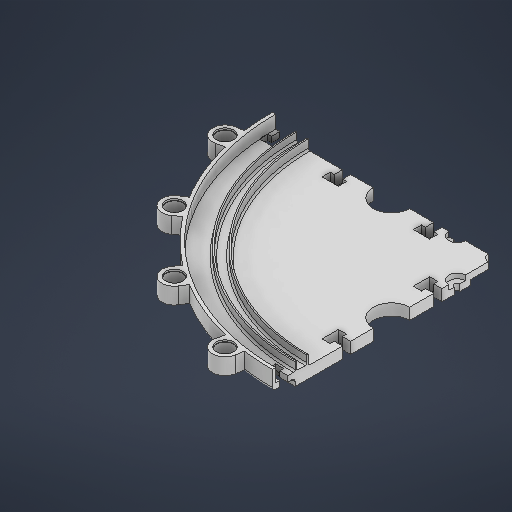
# Autodesk Inventor part: Base_frame_v2
Saved by Autodesk Inventor 2026 (Build 300175050, 175E)
## iProperties
Created: 2026-04-30
Part Number: Base_frame_v2
Material: Generic
Document SubType Name: Modeling
Designer: sniel
Density: 1 g/cm^3
Appearance: Default
Author: sniel
Autodesk Inventor part; units mm, degrees
ref_plane "YZ Plane" through (0, 0, 0) normal (1, 0, 0) x (0, 1, 0)
ref_plane "XZ Plane" through (0, 0, 0) normal (0, 1, 0) x (-1, 0, 0)
ref_plane "XY Plane" through (0, 0, 0) normal (0, 0, 1) x (1, 0, 0)
sketch "Sketch1" plane through (0, 0, 0) normal (1, 0, 0) x (0, 1, 0)
  line L0 (0, 122.235526) -> (11, 122.235526)
  line L1 (5, 0) -> (0, 0)
  line L2 (11, 122.235526) -> (11, 114.235526)
  line L3 (5, 0) -> (5, 114.235526)
  line L4 (11, 118.235526) -> (11, 115.085526)
  line L5 (11, 118.235526) -> (11, 121.385526)
  line L6 (11, 118.235526) -> (6, 118.235526)
  line L7 (6, 118.235526) -> (6, 115.085526)
  line L8 (6, 115.085526) -> (11, 115.085526)
  line L9 (6, 118.235526) -> (6, 121.385526)
  line L10 (6, 121.385526) -> (11, 121.385526)
  line L11 (5, 0) -> (-2, 0)
  line L12 (-2, 0) -> (-2, 122.235526)
  line L13 (-2, 122.235526) -> (0, 122.235526)
  line L14 (5, 114.235526) -> (11, 114.235526)
  line L15 (11, 118.235526) -> (12, 118.235526)
  line L16 (12, 118.235526) -> (12, 134.235526)
  line L17 (6, 118.235526) -> (6, 134.235526)
  line L18 (6, 134.235526) -> (12, 134.235526)
  line L19 (12, 134.235526) -> (14, 134.235526)
  line L20 (14, 134.235526) -> (14, 136.235526)
  line L21 (6, 118.235526) -> (2.5, 118.235526)
  line L22 (2.5, 118.235526) -> (2.5, 134.235526)
  line L23 (2.5, 134.235526) -> (2.5, 136.235526)
  line L24 (2.5, 136.235526) -> (14, 136.235526)
  point P0 (2.5, 122.235526)
  point P1 (6, 122.235526)
  dimension "d0" = 8
  dimension "d1" = 3.15
  dimension "d2" = 3.15
  dimension "d3" = 5
  dimension "d12" = 7
  dimension "d16" = 1
  dimension "d17" = 16
  dimension "d18" = 16
  dimension "d19" = 2
  dimension "d20" = 2
  dimension "d21" = 3.5
  dimension "d22" = 16
  dimension "d23" = 2
  constraints: 50 end point, 4 horizontal, 4 perpendicular, 4 point on line, 3 vertical, 1 midpoint
  measures "d0" distance of L0.end L2.end
  measures "d1" distance of L4.start L4.end
  measures "d2" distance of L4.start L5.end
  measures "d3" distance of L4.start L6.end
  measures "d12" distance of L1.start L11.end
  measures "d16" distance of L4.start L15.end
  measures "d17" distance of L15.end L16.end
  measures "d18" distance of L6.end L17.end
  measures "d19" distance of L16.end L19.end
  measures "d20" distance of L19.end L20.end
  measures "d21" distance of L6.end L21.end
  measures "d22" distance of L21.end L22.end
  measures "d23" distance of L22.end L23.end
revolve "Revolution1" add sketch "Sketch1" angle 360 about axis through (0, 5, 0) along (0, -1, 0) contours L0 L22 L21 L7 L8 L2 L14 L3 L1 L11 L12 L13 | L22 L23 L24 L20 L19 L18 L17 L0 | L0 L17 L9 L21 L22 | L0 L2 L10 L17
sketch "Sketch5" plane through (0, 5, 0) normal (0, 1, 0) x (1, 0, 0)
  circle A0 centre (0, 0) radius 4.1
  line L0 (0, 0) -> (0, -63.331)
  line L1 (0, 0) -> (-63.331, 0)
  circle A1 centre (0, -63.331) radius 11.1
  circle A2 centre (-63.331, 0) radius 11.1
  line L2 (0, 0) -> (0, 63.331)
  circle A3 centre (0, 63.331) radius 11.1
  line L3 (0, 0) -> (0, 35)
  line L4 (0, 35) -> (0, 37.5)
  line L5 (0, 35) -> (0, 32.5)
  line L6 (0, 32.5) -> (-5, 32.5)
  line L7 (-5, 32.5) -> (-5, 30)
  line L8 (-5, 30) -> (-10, 30)
  line L9 (-10, 30) -> (-10, 40)
  line L10 (-10, 40) -> (-5, 40)
  line L11 (-5, 40) -> (-5, 37.5)
  line L12 (-5, 37.5) -> (0, 37.5)
  line L13 (0, 0) -> (-132, 132)
  line L14 (0, 0) -> (186.67619, 0) construction
  line L15 (-32.5, 0) -> (-32.5, 5)
  line L16 (-32.5, 5) -> (-30, 5)
  line L17 (-30, 5) -> (-30, 10)
  line L18 (-30, 10) -> (-40, 10)
  line L19 (-40, 10) -> (-40, 5)
  line L20 (-40, 5) -> (-37.5, 5)
  line L21 (-37.5, 5) -> (-37.5, 0)
  line L22 (0, 0) -> (-178, 0)
  line L23 (0, -32.5) -> (-5, -32.5)
  line L24 (-5, -32.5) -> (-5, -30)
  line L25 (-5, -30) -> (-10, -30)
  line L26 (-10, -30) -> (-10, -40)
  line L27 (-10, -40) -> (-5, -40)
  line L28 (-5, -37.5) -> (0, -37.5)
  line L29 (-40, -10) -> (-40, -5)
  line L30 (-40, -5) -> (-37.5, -5)
  line L31 (-32.5, -5) -> (-30, -5)
  line L32 (-30, -5) -> (-30, -10)
  line L33 (-32.5, 0) -> (-32.5, -5)
  line L34 (-30, -10) -> (-40, -10)
  line L35 (-37.5, -5) -> (-37.5, 0)
  line L36 (-5, -37.5) -> (-5, -40)
  line L37 (0, -63.331) -> (0, -88.331)
  line L38 (-10, -85.831) -> (-10, -95.831)
  line L39 (-10, -95.831) -> (-5, -95.831)
  line L40 (0, -88.331) -> (-5, -88.331)
  line L41 (-5, -88.331) -> (-5, -85.831)
  line L42 (-5, -93.331) -> (0, -93.331)
  line L43 (-5, -85.831) -> (-10, -85.831)
  line L44 (-5, -93.331) -> (-5, -95.831)
  line L45 (-63.331, 0) -> (-88.331, 0)
  line L46 (-85.831, -5) -> (-85.831, -10)
  line L47 (-88.331, -5) -> (-85.831, -5)
  line L48 (-88.331, 0) -> (-88.331, -5)
  line L49 (-93.331, -5) -> (-93.331, 0)
  line L50 (-85.831, -10) -> (-95.831, -10)
  line L51 (-95.831, -10) -> (-95.831, -5)
  line L52 (-95.831, -5) -> (-93.331, -5)
  line L53 (0, -88.331) -> (0, -93.331)
  line L54 (-93.331, 0) -> (-88.331, 0)
  point P0 (-37.5, 0)
  point P1 (-37.5, 0)
  point P2 (0, -37.5)
  dimension "d13" = 8.2
  dimension "d32" = 63.331
  dimension "d33" = 63.331
  dimension "d34" = 22.2
  dimension "d35" = 22.2
  dimension "d36" = 63.331
  dimension "d37" = 22.2
  dimension "d44" = 35
  dimension "d45" = 2.5
  dimension "d46" = 2.5
  dimension "d47" = 5
  dimension "d48" = 2.5
  dimension "d49" = 10
  dimension "d50" = 5
  dimension "d51" = 135
  dimension "d52" = 25
  dimension "d53" = 25
  constraints: 110 end point, 22 symmetric about line, 16 point on line, 6 perpendicular, 6 vertical, 4 centre point, 4 coincident, 3 horizontal, 1 equal length
  measures "d13" diameter of A0
  measures "d32" distance of L0.start L0.end
  measures "d33" distance of L0.start L1.end
  measures "d34" diameter of A1
  measures "d35" diameter of A2
  measures "d36" distance of L0.start L2.end
  measures "d37" diameter of A3
  measures "d44" distance of L0.start L3.end
  measures "d45" distance of L3.end L4.end
  measures "d46" distance of L3.end L5.end
  measures "d47" distance of L5.end L6.end
  measures "d48" distance of L6.end L7.end
  measures "d49" distance of L8.end L9.end
  measures "d50" distance of L9.end L10.end
  measures "d51" angle of L14 L13
  measures "d52" distance of L37.start L37.end
  measures "d53" distance of L45.start L45.end
extrude "Extrusion4" cut sketch "Sketch5" against normal blind 10
sketch "Sketch2" plane through (0, 0, 0) normal (1, 0, 0) x (0, 1, 0)
  line L0 (88, 190) -> (-72, 190)
  line L1 (-72, 190) -> (-72, -189)
  line L2 (-72, -189) -> (88, -189)
  line L3 (88, -189) -> (88, 190)
  point P0 (0, 0)
  constraints: 8 end point, 2 parallel, 1 horizontal, 1 perpendicular
extrude "Extrusion1" cut sketch "Sketch2" along normal blind 183.5
sketch "Sketch3" plane through (0, 0, 0) normal (0, 0, 1) x (1, 0, 0)
  line L0 (129, 60) -> (-156, 60)
  line L1 (-156, 60) -> (-156, -67)
  line L2 (-156, -67) -> (129, -67)
  line L3 (129, -67) -> (129, 60)
  point P0 (0, 0)
  constraints: 8 end point, 2 parallel, 1 horizontal, 1 perpendicular
extrude "Extrusion2" cut sketch "Sketch3" against normal blind 183.5
fillet "Fillet1" radius 2 2 edges at (-96.3331, 2.5, 96.3331) (-86.4336, 2.5, 86.4336)
sketch "Sketch6" plane through (0, 5, 0) normal (0, 1, 0) x (0.7071068, 0, -0.7071068)
  circle A0 centre (-16.425, -16.425) radius 1.75
  circle A1 centre (16.425, 16.425) radius 1.75
  arc A2 (-2.899138, 2.899138) -> (-2.899138, -2.899138) centre (0, 0) ccw
  line L0 (0, 0) -> (-79, 0)
  circle A3 centre (-16.425, 16.425) radius 1.75
  constraints: 3 centre point, 2 end point, 1 horizontal, 1 symmetric about line, 1 other
extrude "Extrusion5" cut sketch "Sketch6" against normal blind 10 contours A0 | A3
sketch "Sketch7" plane through (0, -2, 0) normal (0, -1, 0) x (0.7071068, 0, -0.7071068)
  circle A0 centre (0, 0) radius 3.925
  circle A1 centre (0, 0) radius 14.875
  circle A2 centre (0, 0) radius 15.1
  point P0 (0, 0)
  dimension "d63" = 30.2
  constraints: 3 centre point, 1 coincident
  measures "d63" diameter of A2
extrude "Extrusion6" cut sketch "Sketch7" against normal blind 3 contours A1 | A2
sketch "Sketch8" plane through (0, 5, 0) normal (0, 1, 0) x (0.7071068, 0, -0.7071068)
  circle A0 centre (-16.425, -16.425) radius 1.75
  circle A1 centre (-16.425, -16.425) radius 5
  line L0 (0, 0) -> (-57, 0)
  circle A2 centre (-16.425, 16.425) radius 1.75
  circle A3 centre (-16.425, 16.425) radius 5
  dimension "d29" = 10
  constraints: 4 centre point, 2 coincident, 2 end point, 2 symmetric about line, 1 horizontal, 2 other
  measures "d29" diameter of A1
extrude "Extrusion7" cut sketch "Sketch8" against normal blind 3 contours A0 | A1 | A2 | A3
sketch "Sketch9" plane through (0, 14, 0) normal (0, 1, 0) x (0.7071068, 0, -0.7071068)
  line L0 (-133.82283, 25.525844) -> (0, 0)
  line L1 (-112.676528, 76.577533) -> (0, 0)
  arc A0 (-96.333064, 96.333064) -> (-96.333064, -96.333064) centre (0, 0) ccw
  line L2 (-133.82283, 25.525844) -> (-143.645733, 27.3995)
  line L3 (-112.676528, 76.577533) -> (-120.947244, 82.198499)
  circle A1 centre (-138.734281, 26.462672) radius 5
  circle A2 centre (-116.811886, 79.388016) radius 5
  circle A3 centre (-116.811886, 79.388016) radius 7.5
  circle A4 centre (-138.734281, 26.462672) radius 7.5
  line L4 (-139.943419, 19.060781) -> (-135.007021, 18.254395)
  line L5 (-137.133926, 33.789941) -> (-132.247295, 32.722647)
  line L6 (-112.432948, 85.476933) -> (-108.372186, 82.556573)
  line L7 (-120.861425, 73.075233) -> (-116.651364, 70.374553)
  line L8 (0, 0) -> (-202, 0)
  line L9 (-133.82283, -25.525844) -> (0, 0)
  line L10 (-112.676528, -76.577533) -> (0, 0)
  arc A5 (-96.333064, 96.333064) -> (-96.333064, -96.333064) centre (0, 0) ccw
  line L11 (-133.82283, -25.525844) -> (-143.645733, -27.3995)
  line L12 (-112.676528, -76.577533) -> (-120.947244, -82.198499)
  circle A6 centre (-138.734281, -26.462672) radius 5
  circle A7 centre (-116.811886, -79.388016) radius 5
  circle A8 centre (-116.811886, -79.388016) radius 7.5
  circle A9 centre (-138.734281, -26.462672) radius 7.5
  line L13 (-139.943419, -19.060781) -> (-135.007021, -18.254395)
  line L14 (-137.133926, -33.789941) -> (-132.247295, -32.722647)
  line L15 (-112.432948, -85.476933) -> (-108.372186, -82.556573)
  line L16 (-120.861425, -73.075233) -> (-116.651364, -70.374553)
  point P0 (-116.651364, -70.374553)
  point P1 (-135.007021, -18.254395)
  dimension "d38" = 10
  dimension "d39" = 10
  dimension "d40" = 15
  dimension "d41" = 15
  constraints: 34 end point, 22 point on circle, 18 symmetric about line, 5 centre point, 4 coincident, 4 point on line, 4 tangent, 3 horizontal, 2 midpoint, 15 other
  measures "d38" distance of L0.start L2.end
  measures "d39" distance of L1.start L3.end
  measures "d40" diameter of A3
  measures "d41" diameter of A4
extrude "Extrusion8" add sketch "Sketch9" against normal blind 10 contours A0 A4 | A4 L5 A0 | A0 L4 A4 | L7 A3 A0 | A0 A3 | A0 A9 L13 | A0 A9 | A0 A8 | A8 L16 A0 | A3 L6 A0 | A0 L14 A9 | A0 L15 A8
sketch "Sketch10" plane through (-134.235526, 2.5, 0) normal (0, -1, 0) x (1, 0, 0)
  line L0 (129.235526, 93.331) -> (134.235526, 93.331)
  line L1 (129.235526, 95.831) -> (129.235526, 93.331)
  line L2 (124.235526, 95.831) -> (129.235526, 95.831)
  line L3 (124.235526, 85.831) -> (124.235526, 95.831)
  line L4 (134.235526, 88.331) -> (129.235526, 88.331)
  line L5 (129.235526, 85.831) -> (124.235526, 85.831)
  line L6 (129.235526, 88.331) -> (129.235526, 85.831)
  line L7 (134.235526, 134.235526) -> (134.235526, 122.235526)
  line L8 (134.235526, 134.235526) -> (134.235526, 131.735526)
  line L9 (129.235526, 131.735526) -> (134.235526, 131.735526)
  line L10 (129.235526, 134.235526) -> (129.235526, 131.735526)
  line L11 (124.235526, 134.235526) -> (129.235526, 134.235526)
  line L12 (124.235526, 124.235526) -> (124.235526, 134.235526)
  line L13 (134.235526, 126.735526) -> (129.235526, 126.735526)
  line L14 (129.235526, 124.235526) -> (124.235526, 124.235526)
  line L15 (129.235526, 126.735526) -> (129.235526, 124.235526)
  arc A0 (134.235526, 14.875) -> (119.360526, 0) centre (134.235526, 0) ccw
  line L16 (134.235526, 14.875) -> (134.235526, 21.478458)
  arc A1 (134.235526, 24.978458) -> (134.235526, 21.478458) centre (134.235526, 23.228458) ccw
  line L17 (134.235526, 24.978458) -> (134.235526, 32.5)
  line L18 (134.235526, 32.5) -> (129.235526, 32.5)
  line L19 (129.235526, 32.5) -> (129.235526, 30)
  line L20 (129.235526, 30) -> (124.235526, 30)
  line L21 (124.235526, 30) -> (124.235526, 40)
  line L22 (124.235526, 40) -> (129.235526, 40)
  line L23 (129.235526, 40) -> (129.235526, 37.5)
  line L24 (129.235526, 37.5) -> (134.235526, 37.5)
  line L25 (134.235526, 37.5) -> (134.235526, 52.231)
  arc A2 (134.235526, 74.431) -> (134.235526, 52.231) centre (134.235526, 63.331) ccw
  line L26 (134.235526, 74.431) -> (134.235526, 88.331)
  line L27 (134.235526, 88.331) -> (129.235526, 88.331)
  line L28 (129.235526, 88.331) -> (129.235526, 85.831)
  line L29 (129.235526, 85.831) -> (124.235526, 85.831)
  line L30 (124.235526, 85.831) -> (124.235526, 95.831)
  line L31 (124.235526, 95.831) -> (129.235526, 95.831)
  line L32 (129.235526, 95.831) -> (129.235526, 93.331)
  line L33 (129.235526, 93.331) -> (134.235526, 93.331)
  line L34 (134.235526, 93.331) -> (134.235526, 122.235526)
  arc A3 (134.235526, 122.235526) -> (12, 0) centre (134.235526, 0) ccw
  line L35 (12, 0) -> (40.904526, 0)
  line L36 (40.904526, 0) -> (40.904526, 5)
  line L37 (40.904526, 5) -> (38.404526, 5)
  line L38 (38.404526, 5) -> (38.404526, 10)
  line L39 (38.404526, 10) -> (48.404526, 10)
  line L40 (48.404526, 10) -> (48.404526, 5)
  line L41 (48.404526, 5) -> (45.904526, 5)
  line L42 (45.904526, 5) -> (45.904526, 0)
  line L43 (45.904526, 0) -> (59.804526, 0)
  arc A4 (82.004526, 0) -> (59.804526, 0) centre (70.904526, 0) ccw
  line L44 (82.004526, 0) -> (96.735526, 0)
  line L45 (96.735526, 0) -> (96.735526, 5)
  line L46 (96.735526, 5) -> (94.235526, 5)
  line L47 (94.235526, 5) -> (94.235526, 10)
  line L48 (94.235526, 10) -> (104.235526, 10)
  line L49 (104.235526, 10) -> (104.235526, 5)
  line L50 (104.235526, 5) -> (101.735526, 5)
  line L51 (101.735526, 5) -> (101.735526, 0)
  line L52 (101.735526, 0) -> (119.360526, 0)
  line L53 (2.5, 0) -> (2.5, 5)
  line L54 (2.5, 5) -> (0, 5)
  line L55 (0, 5) -> (0, 10)
  line L56 (0, 10) -> (10, 10)
  line L57 (10, 10) -> (10, 5)
  line L58 (10, 5) -> (7.5, 5)
  line L59 (7.5, 5) -> (7.5, 0)
  arc A5 (134.235526, 134.235526) -> (0, 0) centre (134.235526, 0) ccw
  line L60 (0, 0) -> (2.5, 0)
  line L61 (0, 0) -> (10, 0)
  point P0 (129.235526, 134.142374)
  point P1 (124.235526, 133.862528)
  point P2 (0.372998, 10)
  point P3 (0.093152, 5)
  point P4 (2.5, 0)
  point P5 (7.5, 0)
  dimension "d54" = 2.5
  dimension "d55" = 2.5
  constraints: 122 end point, 10 centre point, 10 point on circle, 2 point on line
  measures "d54" distance of L7.start L8.end
  measures "d55" distance of L60.start L60.end
extrude "Extrusion9" cut sketch "Sketch10" against normal up to surface (3.5 mm away) contours L7 L13 L15 L14 L12 A5 L10 L9 | A5 L12 L11 L10 | L53 L54 A5 L56 L57 L58 L59 L61 | L54 L55 L56 A5
fillet "Fillet2" radius 1 4 edges at (-85.8325, 6, 85.8325) (-81.3778, 6, 81.3778) (-86.4336, 6, 86.4336) (-80.7767, 5, 80.7767)
sketch "Sketch11" plane through (-95.831, -2, 10) normal (0, -1, 0) x (1, 0, 0)
  line L0 (95.831, 5.1) -> (95.831, 11.478458)
  arc A0 (95.831, 14.978458) -> (95.831, 11.478458) centre (95.831, 13.228458) ccw
  line L1 (95.831, 14.978458) -> (95.831, 22.5)
  line L2 (95.831, 22.5) -> (90.831, 22.5)
  line L3 (90.831, 22.5) -> (90.831, 20)
  line L4 (90.831, 20) -> (85.831, 20)
  line L5 (85.831, 20) -> (85.831, 30)
  line L6 (85.831, 30) -> (90.831, 30)
  line L7 (90.831, 30) -> (90.831, 27.5)
  line L8 (90.831, 27.5) -> (95.831, 27.5)
  line L9 (95.831, 27.5) -> (95.831, 42.231)
  arc A1 (95.831, 64.431) -> (95.831, 42.231) centre (95.831, 53.331) ccw
  line L10 (95.831, 64.431) -> (95.831, 78.331)
  line L11 (95.831, 78.331) -> (90.831, 78.331)
  line L12 (90.831, 78.331) -> (90.831, 75.831)
  line L13 (90.831, 75.831) -> (85.831, 75.831)
  line L14 (85.831, 75.831) -> (85.831, 85.831)
  line L15 (85.831, 85.831) -> (90.831, 85.831)
  line L16 (90.831, 85.831) -> (90.831, 83.331)
  line L17 (90.831, 83.331) -> (95.831, 83.331)
  line L18 (95.831, 83.331) -> (95.831, 112.235526)
  arc A2 (95.831, 112.235526) -> (-26.404526, -10) centre (95.831, -10) ccw
  line L19 (-26.404526, -10) -> (2.5, -10)
  line L20 (2.5, -10) -> (2.5, -5)
  line L21 (2.5, -5) -> (0, -5)
  line L22 (0, -5) -> (0, 0)
  line L23 (0, 0) -> (10, 0)
  line L24 (10, 0) -> (10, -5)
  line L25 (10, -5) -> (7.5, -5)
  line L26 (7.5, -5) -> (7.5, -10)
  line L27 (7.5, -10) -> (21.4, -10)
  arc A3 (43.6, -10) -> (21.4, -10) centre (32.5, -10) ccw
  line L28 (43.6, -10) -> (58.331, -10)
  line L29 (58.331, -10) -> (58.331, -5)
  line L30 (58.331, -5) -> (55.831, -5)
  line L31 (55.831, -5) -> (55.831, 0)
  line L32 (55.831, 0) -> (65.831, 0)
  line L33 (65.831, 0) -> (65.831, -5)
  line L34 (65.831, -5) -> (63.331, -5)
  line L35 (63.331, -5) -> (63.331, -10)
  line L36 (63.331, -10) -> (70.852542, -10)
  line L37 (95.831, 53.331) -> (32.5, 53.331)
  line L38 (32.5, -10) -> (32.5, 53.331)
  line L39 (27.5, 58.331) -> (37.5, 58.331)
  line L40 (37.5, 58.331) -> (37.5, 48.331)
  line L41 (37.5, 48.331) -> (27.5, 48.331)
  line L42 (27.5, 48.331) -> (27.5, 58.331)
  line L43 (27.5, 58.331) -> (37.5, 48.331) construction
  line L44 (37.5, 58.331) -> (27.5, 48.331) construction
  arc A4 (95.831, 5.1) -> (80.731, -10) centre (95.831, -10) ccw
  arc A5 (74.352542, -10) -> (70.852542, -10) centre (72.602542, -10) ccw
  line L45 (74.352542, -10) -> (80.731, -10)
  dimension "d59" = 10
  dimension "d60" = 10
  constraints: 16 end point, 2 horizontal, 2 midpoint, 2 parallel, 1 perpendicular, 1 vertical
  measures "d59" distance of L40.end L41.end
  measures "d60" distance of L39.end L40.end
extrude "Extrusion10" cut sketch "Sketch11" against normal blind 5 contours L40 L41 L38 L37 | L37 L38 L41 L42 L39 L40
sketch "Sketch12" plane through (0, 14, 0) normal (0, 1, 0) x (0.7071068, 0, -0.7071068)
  circle A0 centre (-138.734281, 26.462672) radius 5
  circle A1 centre (-116.811886, -79.388016) radius 5
  circle A2 centre (-116.811886, 79.388016) radius 5
  circle A3 centre (-138.734281, -26.462672) radius 5
  line L0 (-132.247295, 32.722647) -> (-137.133926, 33.789941)
  arc A4 (-137.133926, 33.789941) -> (-139.943419, 19.060781) centre (-138.734281, 26.462672) ccw
  line L1 (-139.943419, 19.060781) -> (-135.007021, 18.254395)
  arc A5 (-135.007021, 18.254395) -> (-135.007021, -18.254395) centre (0, 0) ccw
  line L2 (-135.007021, -18.254395) -> (-139.943419, -19.060781)
  arc A6 (-139.943419, -19.060781) -> (-137.133926, -33.789941) centre (-138.734281, -26.462672) ccw
  line L3 (-137.133926, -33.789941) -> (-132.247295, -32.722647)
  arc A7 (-132.247295, -32.722647) -> (-116.651364, -70.374553) centre (0, 0) ccw
  line L4 (-116.651364, -70.374553) -> (-120.861425, -73.075233)
  arc A8 (-120.861425, -73.075233) -> (-112.432948, -85.476933) centre (-116.811886, -79.388016) ccw
  line L5 (-112.432948, -85.476933) -> (-108.372186, -82.556573)
  arc A9 (-108.372186, -82.556573) -> (-96.333064, -96.333064) centre (0, 0) ccw
  line L6 (-96.333064, -96.333064) -> (-94.918851, -94.918851)
  arc A10 (-94.918851, 94.918851) -> (-94.918851, -94.918851) centre (0, 0) ccw
  line L7 (-94.918851, 94.918851) -> (-96.333064, 96.333064)
  arc A11 (-96.333064, 96.333064) -> (-108.372186, 82.556573) centre (0, 0) ccw
  line L8 (-108.372186, 82.556573) -> (-112.432948, 85.476933)
  arc A12 (-112.432948, 85.476933) -> (-120.861425, 73.075233) centre (-116.811886, 79.388016) ccw
  line L9 (-120.861425, 73.075233) -> (-116.651364, 70.374553)
  arc A13 (-116.651364, 70.374553) -> (-132.247295, 32.722647) centre (0, 0) ccw
  circle A14 centre (-116.811886, -79.388016) radius 5.25
  circle A15 centre (-138.734281, -26.462672) radius 5.25
  circle A16 centre (-138.734281, 26.462672) radius 5.25
  circle A17 centre (-116.811886, 79.388016) radius 5.25
  dimension "d64" = 10.5
  dimension "d65" = 10.5
  dimension "d66" = 10.5
  dimension "d67" = 10.5
  constraints: 4 centre point, 4 coincident
  measures "d64" diameter of A14
  measures "d65" diameter of A15
  measures "d66" diameter of A16
  measures "d67" diameter of A17
extrude "Extrusion11" cut sketch "Sketch12" against normal blind 1 contours A0 | A2 | A3 | A14 | A15 | A16 | A17
body "Solid1"
